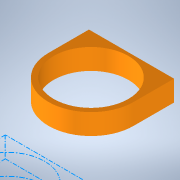
# Autodesk Inventor part: XPS-Hinten
Saved by Autodesk Inventor 2020.3 (Build 243373010, 373A)
## iProperties
Created: 2020-10-19
Part Number: XPS-Hinten
Material: Generisch
Document SubType Name: Modeling
Designer: Stefan
Density: 1 g/cm^3
Appearance: Vorgabe
Author: Stefan
Autodesk Inventor part; units mm, degrees
ref_plane "YZ Plane" through (0, 0, 0) normal (1, 0, 0) x (0, 1, 0)
ref_plane "XZ Plane" through (0, 0, 0) normal (0, 1, 0) x (-1, 0, 0)
ref_plane "XY Plane" through (0, 0, 0) normal (0, 0, 1) x (1, 0, 0)
sketch "Skizze1" plane through (0, 0, 0) normal (0, 0, 1) x (1, 0, 0)
  line L0 (-240.4724, 39.0464) -> (579.5276, 39.0464)
  line L1 (579.5276, 39.0464) -> (579.5276, -160.9536)
  line L2 (579.5276, -160.9536) -> (-240.4724, -160.9536)
  line L3 (-240.4724, -160.9536) -> (-240.4724, 39.0464)
  point P0 (0, 0)
  dimension "d0" = 200
  dimension "d1" = 820
  constraints: 8 end point, 2 parallel, 1 horizontal, 1 perpendicular
  measures "d0" distance of L0.end L1.end
  measures "d1" distance of L1.end L2.end
extrude "Extrusion1" add sketch "Skizze1" along normal blind 800
fillet "Rundung1" radius 410 2 edges at (-240.4724, -60.9536, 800) (579.5276, -60.9536, 800)
sketch "Skizze2" plane through (-240.4724, -160.9536, 0) normal (0, -1, 0) x (1, 0, 0)
  circle A0 centre (410, 390) radius 360
  line L0 (820, 0) -> (820, 390) projected
  line L1 (0, 0) -> (820, 0) projected
  point P0 (240.4724, 0)
  dimension "d5" = 720
  dimension "d6" = 410
  dimension "d7" = 390
  constraints: 1 centre point
  measures "d5" diameter of A0
  measures "d6" distance from line of L0 A0.centre
  measures "d7" distance from line of L1 A0.centre
extrude "Extrusion2" cut sketch "Skizze2" against normal up to surface (200 mm away)
